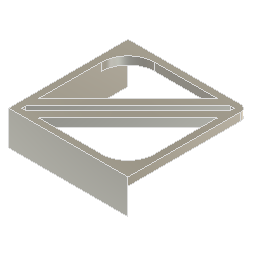
Нахождение центра с краев (Autodesk Fusion 360 design; units mm, degrees)
Autodesk Fusion 360 part; units mm, degrees
sketch "Sketch1" plane through (0, 0, 0) normal (0, 0, 1) x (1, 0, 0)
  line L0 (-20, -20) -> (10, -20)
  line L1 (20, -10) -> (20, 20)
  line L2 (20, 20) -> (-10, 20)
  line L3 (-20, 10) -> (-20, -20)
  line L4 (-22.5, -22.5) -> (22.5, -22.5)
  line L5 (22.5, -22.5) -> (22.5, 22.5)
  line L6 (22.5, 22.5) -> (-22.5, 22.5)
  line L7 (-22.5, 22.5) -> (-22.5, -22.5)
  line L8 (-20, 20) -> (-22.5, 22.5)
  line L9 (20, -20) -> (22.5, -22.5)
  line L10 (-13.636, -20) -> (22.5, 16.136)
  line L11 (-20, -13.636) -> (16.136, 22.5)
  line L12 (-22.5, -22.5) -> (22.5, 22.5)
  line L13 (-21.7929, -23.2071) -> (23.2071, 21.7929)
  line L14 (-23.2071, -21.7929) -> (21.7929, 23.2071)
  arc A0 (10, -20) -> (20, -10) centre (10, -10) ccw
  arc A1 (-10, 20) -> (-20, 10) centre (-10, 10) ccw
  line L15 (20, -20) -> (10, -20)
  line L16 (-20, 20) -> (-20, 10)
  dimension "d1" = 45
  dimension "d2" = 45
  dimension "d11" = 1
  dimension "d12" = -1
  dimension "d15" = 10
  constraint horizontal L0
  constraint perpendicular L0 L1
  constraint parallel L0 L2
  constraint parallel L1 L3
  constraint horizontal L4
  constraint perpendicular L4 L5
  constraint parallel L4 L6
  constraint parallel L5 L7
  constraint parallel L8 L9
  constraint coincident L6 L11.end
  constraint coincident L5 L10.end
  constraint coincident L0 L10.start
  constraint coincident L3 L11.start
  constraint coincident L9.start L0
  constraint coincident L9.start L1
  constraint tangent L0 A0
  constraint tangent L1 A0
  constraint coincident L8.start L3
  constraint coincident L8.start L2
  constraint tangent L3 A1
  constraint tangent L2 A1
  constraint equal A0 A1
  measures "d1" distance of L5.end L6.end
  measures "d2" distance of L4.end L5.end
  measures "d15" radius of A0
extrude "Extrude1" add sketch "Sketch1" along normal blind 3 contours L0 L4 L9 L13 L15 | L0 L1 L10 L13 | L1 L5 L9 L10 A0 L15 | L0 L4 L12 L13 | L1 L5 L10 L13 | L3 L7 L12 L14 | L1 L5 L12 L13 | L3 L7 L8 L14 L16 | L2 L3 L11 L14 | L2 L6 L12 L14 | L2 L6 L11 L14 | L2 L6 L8 L11 A1 L16
extrude "Extrude2" add sketch "Sketch1" against normal blind 10 contours L0 L4 L9 L13 L15 | L0 L4 L12 L13 | L3 L7 L12 L14 | L3 L7 L8 L14 L16
fillet "Fillet1" radius 2.5 1 edges at (22.5, 22.5, 1.5)
